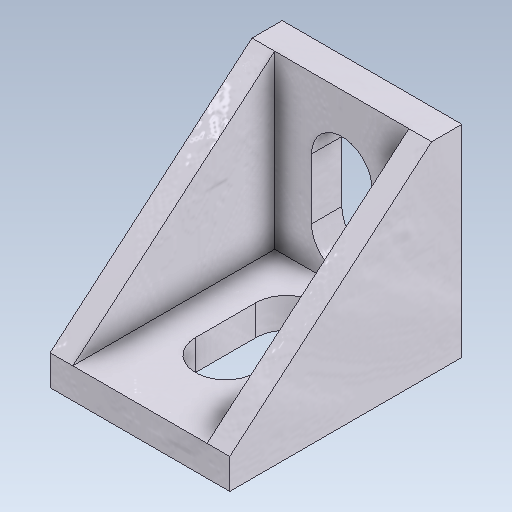
# Autodesk Inventor part: Cast corner bracket-20x20x17
Saved by Autodesk Inventor 2021 (Build 250183000, 183)
## iProperties
Created: 2022-05-23
Part Number: Cast corner bracket-20x20x17
Material: Aluminio 6061, soldado
Document SubType Name: Modeling
Designer: 79449
Density: 2.7 g/cm^3
Appearance: Soldadura - Aluminio
Author: 79449
Autodesk Inventor part; units mm, degrees
ref_plane "YZ Plane" through (0, 0, 0) normal (1, 0, 0) x (0, 1, 0)
ref_plane "XZ Plane" through (0, 0, 0) normal (0, 1, 0) x (-1, 0, 0)
ref_plane "XY Plane" through (0, 0, 0) normal (0, 0, 1) x (1, 0, 0)
sketch "Boceto1" plane through (0, 0, 0) normal (0, 0, 1) x (1, 0, 0)
  line L0 (8.9, -10) -> (-8.9, -10)
  line L1 (-8.9, -10) -> (-8.9, 10)
  line L2 (-8.9, 10) -> (8.9, 10)
  line L3 (8.9, 10) -> (8.9, -10)
  line L4 (8.9, -10) -> (-8.9, 10) construction
  line L5 (-8.9, -10) -> (8.9, 10) construction
  line L6 (0, 10) -> (0, -10)
  line L7 (8.9, 0) -> (-8.9, 0)
  line L8 (0, -3) -> (0, 3) construction
  line L9 (3, -3) -> (3, 3)
  line L10 (-3, 3) -> (-3, -3)
  arc A0 (-3, -3) -> (3, -3) centre (0, -3) ccw
  arc A1 (3, 3) -> (-3, 3) centre (0, 3) ccw
  point P0 (0, 0)
  dimension "d0" = 17.8
  dimension "d1" = 20
  dimension "d2" = 6
  dimension "d3" = 6
  constraints: 24 end point, 7 midpoint, 4 point on circle, 4 tangent, 3 parallel, 2 centre point, 1 horizontal, 1 perpendicular, 1 point on line
  measures "d0" distance of L1.end L2.end
  measures "d1" distance of L0.end L1.end
  measures "d2" distance of L8.start L8.end
  measures "d3" distance between parallel lines of L10 L9
extrude "Extrusión1" add sketch "Boceto1" along normal blind 3 contours L0 L6 A0 L9 L7 L3 | L0 L1 L7 L10 A0 L6 | L7 L9 A1 L6 L2 L3 | L1 L2 L6 A1 L10 L7
sketch "Boceto2" plane through (0, 0, 3) normal (0, 0, 1) x (1, 0, 0)
  line L0 (-8.9, 10) -> (-8.9, -10) projected
  line L1 (-8.9, -10) -> (8.9, -10) projected
  line L2 (-8.9, -7) -> (8.9, -7)
  line L3 (8.9, -7) -> (8.9, -10)
  line L4 (8.9, -10) -> (-8.9, -10)
  line L5 (-8.9, -10) -> (-8.9, -7)
  point P0 (0, 0)
  dimension "d6" = 3
  constraints: 8 end point, 2 parallel, 1 horizontal, 1 perpendicular, 1 point on line
  measures "d6" distance between parallel lines of L1 L2
extrude "Extrusión2" add sketch "Boceto2" along normal blind 20
sketch "Boceto3" plane through (8.9, -10, 0) normal (1, 0, 0) x (0, 0, -1)
  line L0 (-3, 20) -> (-3, 3) projected
  line L1 (-3, 3) -> (-23, 3) projected
  line L2 (-3, 20) -> (-23, 3)
  line L3 (-23, 3) -> (-3, 3)
  line L4 (-3, 3) -> (-3, 20)
  point P0 (0, 10)
  constraints: 6 end point, 1 perpendicular
extrude "Extrusión3" add sketch "Boceto3" against normal blind 2.25
sketch "Boceto4" plane through (-8.9, -10, 0) normal (-1, 0, 0) x (0, 0, 1)
  line L0 (3, 20) -> (23, 3) projected
  line L1 (3, 20) -> (23, 3)
  line L2 (3, 3) -> (23, 3) projected
  line L3 (23, 3) -> (3, 3)
  line L4 (3, 3) -> (3, 20)
  point P0 (0, 10)
  constraints: 6 end point, 2 collinear, 1 perpendicular
extrude "Extrusión4" add sketch "Boceto4" against normal blind 2.25
sketch "Boceto5" plane through (6.65, -7, 23) normal (0, 1, 0) x (1, 0, 0)
  line L0 (-6.65, 23) -> (-6.65, 0)
  line L1 (-15.55, 0) -> (2.25, 0) projected
  line L2 (2.25, 20) -> (2.25, 0) projected
  line L3 (-15.55, 23) -> (-15.55, 0) projected
  line L4 (2.25, 11.5) -> (-15.55, 11.5)
  line L5 (2.25, 23) -> (-15.55, 23) projected
  line L6 (-6.65, 14.5) -> (-6.65, 8.5) construction
  line L7 (-9.65, 14.5) -> (-9.65, 8.5)
  line L8 (-3.65, 8.5) -> (-3.65, 14.5)
  arc A0 (-3.65, 14.5) -> (-9.65, 14.5) centre (-6.65, 14.5) ccw
  arc A1 (-9.65, 8.5) -> (-3.65, 8.5) centre (-6.65, 8.5) ccw
  point P0 (-6.65, 11.5)
  dimension "d13" = 23
  dimension "d14" = 11.5
  dimension "d15" = 6
  dimension "d16" = 6
  constraints: 12 end point, 4 midpoint, 4 point on circle, 4 tangent, 2 centre point, 2 point on line, 1 parallel
  measures "d13" distance between parallel lines of L1 L5
  measures "d14" distance between parallel lines of L5 L4
  measures "d15" distance between parallel lines of L8 L7
  measures "d16" distance of L6.start L6.end
extrude "Extrusión5" cut sketch "Boceto5" against normal through all contours A0 L8 L4 L0 | L0 L4 L7 A0 | L4 L8 A1 L0 | L0 A1 L7 L4
